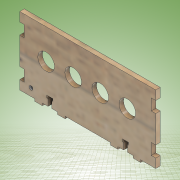
# Autodesk Inventor part: CaraLateral
Saved by Autodesk Inventor 2022 (Build 260153000, 153)
## iProperties
Created: 2022-03-01
Part Number: CaraLateral
Material: Genérico
Document SubType Name: Modeling
Designer: Marco
Density: 1 g/cm^3
Appearance: Valor por defecto
Author: Marco
Autodesk Inventor part; units mm, degrees
ref_plane "YZ Plane" through (0, 0, 0) normal (1, 0, 0) x (0, 1, 0)
ref_plane "XZ Plane" through (0, 0, 0) normal (0, 1, 0) x (-1, 0, 0)
ref_plane "XY Plane" through (0, 0, 0) normal (0, 0, 1) x (1, 0, 0)
sketch "Boceto3" plane through (0, 0, 0) normal (0, 0, 1) x (1, 0, 0)
  line L0 (0, 0) -> (180, 0)
  line L1 (180, 0) -> (180, 90)
  line L2 (180, 90) -> (0, 90)
  line L3 (0, 90) -> (0, 0)
  circle A0 centre (35, 50) radius 11
  circle A1 centre (70.8, 50) radius 11
  circle A2 centre (106.6, 50) radius 11
  circle A3 centre (142.4, 50) radius 11
  circle A4 centre (15, 10) radius 2.5
  dimension "d1" = 90
  dimension "d3" = 22
  dimension "d4" = 50
  dimension "d6" = 35.8
  dimension "d7" = 35.8
  dimension "d8" = 35.8
  dimension "d9" = 35
  dimension "d37" = 5
  dimension "d38" = 10
  dimension "d39" = 15
  dimension "d40" = 180
  constraints: 8 end point, 5 centre point, 3 equal radius, 3 horizontal alignment, 2 parallel, 1 horizontal, 1 perpendicular
  measures "d1" distance of L2.end L0.start
  measures "d3" diameter of A0
  measures "d4" vertical distance of L0.start A0.centre
  measures "d6" distance of A1.centre A0.centre
  measures "d7" distance of A1.centre A2.centre
  measures "d8" distance of A3.centre A2.centre
  measures "d9" horizontal distance of L0.start A0.centre
  measures "d37" diameter of A4
  measures "d38" vertical distance of L0.start A4.centre
  measures "d39" horizontal distance of L0.start A4.centre
  measures "d40" distance of L1.end L2.end
extrude "Extrusión1" add sketch "Boceto3" along normal blind 6
sketch "Boceto4" plane through (0, 0, 6) normal (0, 0, 1) x (1, 0, 0)
  line L0 (36, 12) -> (44, 12)
  line L1 (44, 12) -> (44, 8.9)
  line L2 (36, 8.9) -> (36, 12)
  line L3 (0, 0) -> (180, 0) projected
  line L4 (42.5, 8.9) -> (42.5, 0)
  line L5 (37.5, 0) -> (37.5, 8.9)
  line L6 (44, 8.9) -> (42.5, 8.9)
  line L7 (37.5, 8.9) -> (36, 8.9)
  line L8 (37.5, 0) -> (42.5, 0)
  line L9 (180, 90) -> (0, 90) projected
  line L10 (90, 90) -> (90, 0)
  line L11 (144, 12) -> (136, 12)
  line L12 (136, 12) -> (136, 8.9)
  line L13 (144, 8.9) -> (144, 12)
  line L14 (137.5, 8.9) -> (137.5, 0)
  line L15 (142.5, 0) -> (142.5, 8.9)
  line L16 (136, 8.9) -> (137.5, 8.9)
  line L17 (142.5, 8.9) -> (144, 8.9)
  line L18 (142.5, 0) -> (137.5, 0)
  point P0 (40, 12)
  point P1 (40, 0)
  point P2 (140, 12)
  point P3 (140, 0)
  point P4 (137.5, 0)
  point P5 (142.5, 0)
  dimension "d12" = 8
  dimension "d13" = 3.1
  dimension "d14" = 5
  dimension "d15" = 12
  dimension "d16" = 40
  constraints: 34 end point, 10 symmetric about line, 4 midpoint, 4 parallel, 2 horizontal, 2 point on line, 2 vertical alignment, 1 horizontal alignment, 1 perpendicular
  measures "d12" distance of L0.start L0.end
  measures "d13" distance of L0.end L1.end
  measures "d14" distance of L4.end L5.start
  measures "d15" vertical distance of L5.start L0.start
  measures "d16" distance of L3.start point (40, 0)
sketch "Boceto5" plane through (0, 0, 0) normal (0, -1, 0) x (1, 0, 0)
  line L0 (180, 6) -> (0, 6) projected
  line L1 (180, 0) -> (0, 0) projected
  line L2 (30, 6) -> (20, 6)
  line L3 (20, 6) -> (20, 0)
  line L4 (20, 0) -> (30, 0)
  line L5 (30, 0) -> (30, 6)
  line L6 (50, 6) -> (60, 6)
  line L7 (60, 6) -> (60, 0)
  line L8 (60, 0) -> (50, 0)
  line L9 (50, 0) -> (50, 6)
  line L10 (90, 6) -> (90, 0)
  line L11 (150, 6) -> (160, 6)
  line L12 (160, 6) -> (160, 0)
  line L13 (160, 0) -> (150, 0)
  line L14 (150, 0) -> (150, 6)
  line L15 (130, 6) -> (120, 6)
  line L16 (120, 6) -> (120, 0)
  line L17 (120, 0) -> (130, 0)
  line L18 (130, 0) -> (130, 6)
  point P0 (150, 6)
  point P1 (150, 0)
  point P2 (160, 0)
  point P3 (160, 6)
  point P4 (130, 0)
  point P5 (130, 6)
  point P6 (120, 6)
  point P7 (120, 0)
  point P8 (50, 0)
  point P9 (30, 0)
  point P10 (20, 6)
  dimension "d17" = 10
  dimension "d18" = 10
  dimension "d19" = 20
  dimension "d20" = 20
  constraints: 34 end point, 8 symmetric about line, 4 parallel, 4 point on line, 2 horizontal, 2 midpoint, 2 perpendicular
  measures "d17" distance of L4.end L3.end
  measures "d18" distance of L7.end L8.end
  measures "d19" distance of L8.end L4.end
  measures "d20" distance of L1.end L3.end
extrude "Extrusión2" cut sketch "Boceto4" against normal through all
extrude "Extrusión3" add sketch "Boceto5" along normal blind 3 contours L12 L1 L14 L0 | L18 L1 L16 L0 | L7 L1 L9 L0 | L5 L1 L3 L0
sketch "Boceto7" plane through (0, 0, 6) normal (0, 0, 1) x (1, 0, 0)
  line L0 (0, 78) -> (6, 78)
  line L1 (6, 78) -> (6, 63)
  line L2 (6, 63) -> (0, 63)
  line L3 (180, 90) -> (0, 90) projected
  line L4 (0, 90) -> (0, 0) projected
  line L5 (180, 0) -> (180, 90) projected
  line L6 (0, 45) -> (180, 45)
  line L7 (90, 90) -> (90, 0)
  line L8 (60, 0) -> (120, 0) projected
  line L9 (0, 12) -> (6, 12)
  line L10 (6, 12) -> (6, 27)
  line L11 (6, 27) -> (0, 27)
  line L12 (180, 78) -> (174, 78)
  line L13 (174, 78) -> (174, 63)
  line L14 (174, 63) -> (180, 63)
  line L15 (180, 12) -> (174, 12)
  line L16 (174, 12) -> (174, 27)
  line L17 (174, 27) -> (180, 27)
  point P0 (0, 27)
  point P1 (180, 12)
  point P2 (180, 27)
  point P3 (180, 63)
  point P4 (180, 78)
  dimension "d31" = 6
  dimension "d32" = 15
  dimension "d33" = 12
  constraints: 28 end point, 12 symmetric about line, 4 midpoint, 2 point on line, 1 horizontal, 1 parallel, 1 perpendicular
  measures "d31" distance of L1.end L2.end
  measures "d32" distance of L0.end L1.end
  measures "d33" distance of L3.end L0.start
extrude "Extrusión5" cut sketch "Boceto7" against normal through all contours L5 L15 L16 L17 | L11 L10 L9 L4 | L0 L1 L2 L4 | L5 L14 L13 L12
